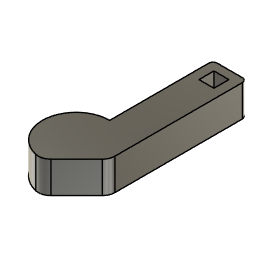
CTS Rubber Band Launcher (Autodesk Fusion 360 design; units mm, degrees)
Autodesk Fusion 360 part; units mm, degrees
sketch "Sketch1" plane through (0, 0, 0) normal (0, 0, 1) x (1, 0, 0)
  line L0 (1.778, -1.778) -> (-1.778, -1.778)
  line L1 (-1.778, -1.778) -> (-1.778, 1.778)
  line L2 (-1.778, 1.778) -> (1.778, 1.778)
  line L3 (1.778, 1.778) -> (1.778, -1.778)
  line L4 (1.778, -1.778) -> (-1.778, 1.778) construction
  line L5 (-1.778, -1.778) -> (1.778, 1.778) construction
  line L6 (0, -1.778) -> (0, -5)
  line L7 (4, -3.778) -> (4, -28.778)
  line L8 (-4, -3.778) -> (-4, -28.778)
  circle A0 centre (-4, -28.778) radius 8
  line L9 (-4, -3.778) -> (4, -3.778)
  line L10 (4, -3.778) -> (4, 3.778)
  line L11 (4, 3.778) -> (-4, 3.778)
  line L12 (-4, 3.778) -> (-4, -3.778)
  line L13 (4, -28.778) -> (-4, -36.778)
  dimension "d1" = 3.556
  dimension "d3" = 4
  dimension "d4" = 4
  dimension "d5" = 25
  dimension "d6" = 25
  dimension "d7" = 2
  dimension "d8" = 2
  constraint horizontal L0
  constraint perpendicular L0 L1
  constraint parallel L0 L2
  constraint parallel L1 L3
  constraint coincident L4 origin
  constraint coincident L5 origin
  constraint midpoint L0 L6.start
  constraint perpendicular L0 L6
  constraint vertical L8
  constraint coincident L8.end A0.centre
  constraint coincident L7.end A0
  constraint perpendicular L7 L9
  constraint perpendicular L9 L10
  constraint perpendicular L10 L11
  constraint perpendicular L9 L12
  constraint coincident A0 L13.end
  measures "d1" distance of L1.end L2.end
  measures "d3" distance of L6 L8
  measures "d4" distance of L6 L7
  measures "d5" distance of L7.start L7.end
  measures "d6" distance of L8.start L8.end
  measures "d7" distance of L0 L9
  measures "d8" distance of L2 L11
extrude "Extrude1" add sketch "Sketch1" along normal blind 7.5 contours L7 L8 A0 L9 | L9 L10 L11 L12 | A0 L13 picked at (0.413, -29.4293)
fillet "Fillet1" radius 3 2 edges at (4, -28.778, 3.75) (-4, -36.778, 3.75)
fillet "Fillet2" radius 1 2 edges at (4, 3.778, 3.75) (-4, 3.778, 3.75)
